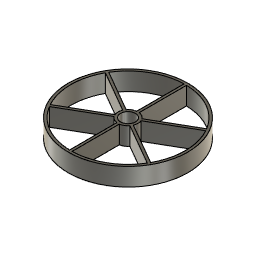
CD CNC wood Storage v2 (Autodesk Fusion 360 design; units mm, degrees)
Autodesk Fusion 360 part; units mm, degrees
sketch "CD Rom Size" plane through (0, 0, 0) normal (0, 0, 1) x (1, 0, 0)
  circle A0 centre (0, 0) radius 7.5
  circle A1 centre (0, 0) radius 7.25
  circle A2 centre (0, 0) radius 60
  circle A3 centre (0, 0) radius 17.5
  dimension "d1" = 15
  dimension "d2" = 14.5
  dimension "d3" = 120
  dimension "d4" = 35
  constraint coincident A0.centre A1.centre
  constraint concentric A0 A1
  constraint concentric A1 A2
  constraint concentric A0 A3
  measures "d1" diameter of A0
  measures "d2" diameter of A1
  measures "d3" diameter of A2
  measures "d4" diameter of A3
extrude "Extrude1" add sketch "CD Rom Size" along normal blind 1.2 contours A2 makes body 1
extrude "Extrude2" add sketch "CD Rom Size" along normal blind 1.19 contours A3 bodies 1
copy_body "CopyPasteBodies1" bodies 1 makes body 2
move_body "Move1" bodies 2 to x (1, 0, 0) y (0, 1, 0) z (0, 0, 1) at (-170, 0, 0)
sketch "Sketch2" plane through (0, 0, 0) normal (0, 0, 1) x (1, 0, 0)
  circle A0 centre (0, 0) radius 60
  circle A1 centre (0, 0) radius 57.5
  line L0 (1.25, -57.5) -> (1.25, 57.5)
  arc A2 (1.25, 57.5) -> (-1.25, 57.5) centre (0, 57.5) ccw
  line L1 (-1.25, 57.5) -> (-1.25, -57.5)
  arc A3 (-1.25, -57.5) -> (1.25, -57.5) centre (0, -57.5) ccw
  line L2 (0, -57.5) -> (0, 57.5) construction
  line L3 (-49.1715, -29.8325) -> (50.4215, 27.6675)
  arc A4 (50.4215, 27.6675) -> (49.1715, 29.8325) centre (49.7965, 28.75) ccw
  arc A5 (-50.4215, -27.6675) -> (-49.1715, -29.8325) centre (-49.7965, -28.75) ccw
  line L4 (49.1715, 29.8325) -> (-50.4215, -27.6675)
  line L5 (50.4215, -27.6675) -> (-49.1715, 29.8325)
  arc A6 (-49.1715, 29.8325) -> (-50.4215, 27.6675) centre (-49.7965, 28.75) ccw
  arc A7 (49.1715, -29.8325) -> (50.4215, -27.6675) centre (49.7965, -28.75) ccw
  line L6 (-50.4215, 27.6675) -> (49.1715, -29.8325)
  dimension "d21" = 115
  dimension "d22" = 120
  dimension "d23" = 2.5
  dimension "d25" = 360
  constraint coincident A0.centre A1.centre
  constraint tangent L0 A2
  constraint tangent A2 L1
  constraint parallel L0 L1
  constraint tangent L1 A3
  constraint tangent L0 A3
  constraint coincident A1 A2.centre
  constraint vertical L2
  constraint coincident A1 A3.centre
  measures "d21" diameter of A1
  measures "d22" diameter of A0
  measures "d23" diameter of A2
extrude "Extrude3" add sketch "Sketch2" along normal blind 18 separate body contours A0 | A1 L3 A4 L4 | A1 L5 A7 L6 | A1 L0 A2 L1 | A1 L0 L1 A3 | A1 L5 A6 L6 | A1 L3 A5 L4 makes body 3
sketch "Sketch3" plane through (0, 0, 0) normal (0, 0, 1) x (1, 0, 0)
  circle A0 centre (0, 0) radius 7.5
  circle A1 centre (0, 0) radius 10
  dimension "d14" = 15
  dimension "d15" = 20
  constraint coincident A0.centre A1.centre
  measures "d14" diameter of A0
  measures "d15" diameter of A1
extrude "Extrude4" add sketch "Sketch3" sketch "Sketch2" along normal blind 18 contours A0 of sketch 2 contours A1 L0 L3 L4 L5 | A1 L0 L3 L5 L6 | A1 L0 L1 L4 L5 | A1 L0 L1 L3 L6 | A1 L1 L4 L5 L6 | A1 L1 L3 L4 L6 bodies 3
extrude "Extrude5" add sketch "Sketch3" along normal blind 18 bodies 3
extrude "Extrude6" cut sketch "Sketch3" along normal blind 18 contours A0 bodies 3
hidden bodies 1 2
equation "d11 = WoodSize"
equation "WoodSize = 18 mm"
equation "d16 = WoodSize"
equation "d18 = WoodSize"
equation "d26 = WoodSize"
